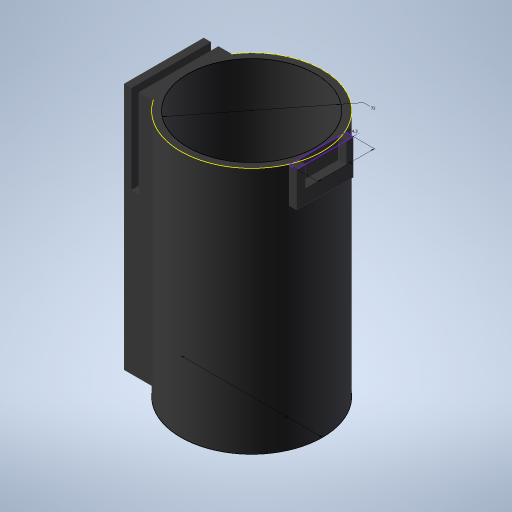
# Autodesk Inventor part: Feeder
Saved by Autodesk Inventor 2023.2 (Build 272271030, 271C)
## iProperties
Created: 2024-03-20
Part Number: Feeder
Material: Generic
Document SubType Name: Modeling
Designer: ryanv
Density: 1 g/cm^3
Appearance: Default
Author: ryanv
Autodesk Inventor part; units mm, degrees
ref_plane "YZ Plane" through (0, 0, 0) normal (1, 0, 0) x (0, 1, 0)
ref_plane "XZ Plane" through (0, 0, 0) normal (0, 1, 0) x (-1, 0, 0)
ref_plane "XY Plane" through (0, 0, 0) normal (0, 0, 1) x (1, 0, 0)
sketch "Sketch1" plane through (0, 0, 0) normal (0, 1, 0) x (-1, 0, 0)
  circle A0 centre (0, 0) radius 40
  dimension "d0" = 80
  constraints: 1 centre point, 1 coincident
  measures "d0" diameter of A0
extrude "Extrusion1" add sketch "Sketch1" along normal blind 140
sketch "Sketch2" plane through (0, 140, 0) normal (0, 1, 0) x (1, 0, 0)
  line L0 (-49, -23) -> (-33, -23)
  line L1 (-33, -23) -> (-33, 22)
  line L2 (-33, 22) -> (-49, 22)
  line L3 (-49, 22) -> (-49, -23)
  point P0 (0, 0)
  constraints: 8 end point, 2 parallel, 1 horizontal, 1 perpendicular
extrude "Extrusion2" add sketch "Sketch2" against normal blind 140
sketch "Sketch3" plane through (0, 140, 0) normal (0, 1, 0) x (1, 0, 0)
  circle A0 centre (0, 0) radius 36
  arc A1 (-33, -22.6053) -> (-33.4066, 22) centre (0, 0) ccw projected
  dimension "d25" = 72
  constraints: 1 centre point, 1 coincident, 1 concentric
  measures "d25" diameter of A0
extrude "Extrusion3" cut sketch "Sketch3" against normal blind 140
sketch "Sketch4" plane through (0, 140, 0) normal (0, 1, 0) x (1, 0, 0)
  line L0 (-45, 25) -> (-40.7, 25)
  line L1 (-40.7, 25) -> (-40.7, -27)
  line L2 (-40.7, -27) -> (-45, -27)
  line L3 (-45, -27) -> (-45, 25)
  line L4 (-49, 22) -> (-49, -23) projected
  point P0 (0, 0)
  dimension "d9" = 4.3
  dimension "d10" = 4
  constraints: 8 end point, 2 parallel, 1 horizontal, 1 perpendicular
  measures "d9" distance between parallel lines of L1 L3
  measures "d10" distance between parallel lines of L3 L4
extrude "Extrusion4" cut sketch "Sketch4" against normal blind 50
sketch "Sketch5" plane through (0, 140, 0) normal (0, 1, 0) x (1, 0, 0)
  line L0 (37.2, -16) -> (41.5, -16)
  line L1 (41.5, -16) -> (41.5, 16)
  line L2 (41.5, 16) -> (37.2, 16)
  line L3 (37.2, 16) -> (37.2, -16)
  point P0 (0, 0)
  point P1 (39.35, -16)
  dimension "d13" = 4.3
  dimension "d14" = 32
  constraints: 8 end point, 2 parallel, 1 horizontal, 1 midpoint, 1 perpendicular
  measures "d13" distance of L2.end L1.end
  measures "d14" distance from line of L2 point (39.35, -16)
extrude "Extrusion5" add sketch "Sketch5" against normal blind 20
sketch "Sketch6" plane through (0, 140, 0) normal (0, 1, 0) x (1, 0, 0)
  line L0 (37, 12) -> (43.2, 12)
  line L1 (43.2, 12) -> (43.2, -11)
  line L2 (43.2, -11) -> (37, -11)
  line L3 (37, -11) -> (37, 12)
  line L4 (41.5, 16) -> (37.2, 16) projected
  line L5 (37.2, -16) -> (41.5, -16) projected
  circle A0 centre (0, 0) radius 36 projected
  point P0 (40.1, 12)
  point P1 (40.1, -11)
  dimension "d28" = 23
  dimension "d29" = 37
  dimension "d30" = 5
  dimension "d31" = 6.2
  constraints: 8 end point, 2 midpoint, 2 parallel, 1 horizontal, 1 perpendicular
  measures "d28" distance between parallel lines of L2 L0
  measures "d29" distance from line of L3 A0.centre
  measures "d30" distance between parallel lines of L5 L2
  measures "d31" distance of L0.start L0.end
extrude "Extrusion6" cut sketch "Sketch6" against normal blind 11.8 contours L0 L1 L2 L3
body "Solid1"
